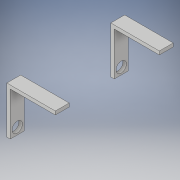
# Autodesk Inventor part: Fixação Caixa de Segurança Dianteira
Saved by Autodesk Inventor 2019 (Build 230136000, 136)
## iProperties
Created: 2020-06-08
Part Number: Fixação Caixa de Segurança Dianteira
Material: Genérico
Document SubType Name: Modeling
Designer: lukas
Density: 1 g/cm^3
Appearance: Padrão
Author: lukas
Autodesk Inventor part; units mm, degrees
ref_plane "YZ Plane" through (0, 0, 0) normal (1, 0, 0) x (0, 1, 0)
ref_plane "XZ Plane" through (0, 0, 0) normal (0, 1, 0) x (-1, 0, 0)
ref_plane "XY Plane" through (0, 0, 0) normal (0, 0, 1) x (1, 0, 0)
sketch "Esboço1" plane through (0, 0, 0) normal (0, 1, 0) x (-1, 0, 0)
  line L0 (0, 0) -> (0, -72)
  line L1 (0, 0) -> (0, -2.5)
  line L2 (0, -72) -> (0, -70.5)
  line L3 (0, -2.5) -> (2, -2.5)
  line L4 (2, -2.5) -> (2, -10.5)
  line L5 (2, -10.5) -> (0, -10.5)
  line L6 (0, -10.5) -> (0, -2.5)
  line L7 (0, -70.5) -> (2, -70.5)
  line L8 (2, -70.5) -> (2, -62.5)
  line L9 (2, -62.5) -> (0, -62.5)
  line L10 (0, -62.5) -> (0, -70.5)
  dimension "d0" = 72
  dimension "d1" = 2.5
  dimension "d2" = 1.5
  dimension "d3" = 2
  dimension "d4" = 8
  dimension "d5" = 2
  dimension "d6" = 8
  constraints: 22 end point, 4 parallel, 2 horizontal, 2 perpendicular, 2 point on line, 1 vertical
  measures "d0" distance of L0.start L0.end
  measures "d1" distance of L0.start L1.end
  measures "d2" distance of L0.end L2.end
  measures "d3" distance of L4.end L5.end
  measures "d4" distance of L3.end L4.end
  measures "d5" distance of L9.end L8.end
  measures "d6" distance of L8.end L7.end
extrude "Extrusão1" add sketch "Esboço1" along normal blind 27
sketch "Esboço2" plane through (0, 0, -2.5) normal (1, 0, 0) x (0, 0, -1)
  line L0 (0, 27) -> (8, 27) projected
  line L1 (8, 0) -> (8, 27) projected
  line L2 (0, 27) -> (8, 27)
  line L3 (8, 27) -> (8, 25)
  line L4 (8, 25) -> (0, 25)
  line L5 (0, 25) -> (0, 27)
  line L6 (68, 27) -> (60, 27) projected
  line L7 (60, 27) -> (68, 27)
  line L8 (68, 27) -> (68, 25)
  line L9 (68, 25) -> (60, 25)
  line L10 (60, 25) -> (60, 27)
  point P0 (-2.5, 0)
  dimension "d9" = 2
  constraints: 16 end point, 4 parallel, 2 horizontal, 2 perpendicular, 2 point on line
  measures "d9" distance of L2.end L3.end
extrude "Extrusão2" add sketch "Esboço2" along normal blind 26
sketch "Esboço3" plane through (0, 0, -2.5) normal (1, 0, 0) x (0, 0, -1)
  line L0 (0, 0) -> (8, 0) projected
  line L1 (4, 0) -> (4, 4)
  line L2 (60, 0) -> (68, 0) projected
  line L3 (64, 0) -> (64, 4)
  circle A0 centre (4, 4) radius 3
  circle A1 centre (64, 4) radius 3
  point P0 (-2.5, 0)
  dimension "d12" = 4
  dimension "d13" = 4
  dimension "d14" = 6
  dimension "d15" = 6
  constraints: 4 end point, 2 centre point, 2 coincident, 2 midpoint, 2 vertical
  measures "d12" distance of L1.start L1.end
  measures "d13" distance of L3.start L3.end
  measures "d14" diameter of A0
  measures "d15" diameter of A1
extrude "Extrusão3" cut sketch "Esboço3" against normal blind 2
